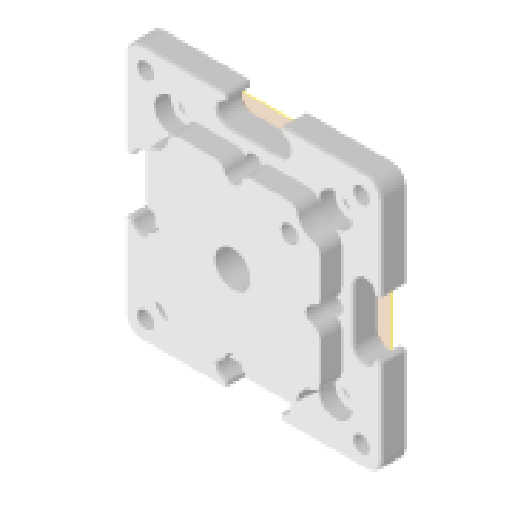
# Autodesk Inventor part: 40_XYZstage_micrometer_motorized_nema8_cube_ontop
Saved by Autodesk Inventor 2024.1 (Build 281209000, 209)
## iProperties
Created: 2023-06-28
Part Number: 40_XYZstage_micrometer_motorized_nema8_cube_ontop
Material: Generisch
Document SubType Name: Modeling
Designer: diederichbenedict
Density: 1 g/cm^3
Appearance: Vorgabe
Author: diederichbenedict
Autodesk Inventor part; units mm, degrees
ref_plane "YZ Plane" through (0, 0, 0) normal (1, 0, 0) x (0, 1, 0)
ref_plane "XZ Plane" through (0, 0, 0) normal (0, 1, 0) x (-1, 0, 0)
ref_plane "XY Plane" through (0, 0, 0) normal (0, 0, 1) x (1, 0, 0)
ref_plane "Arbeitsebene1" through (0, 0, 0) normal (0, 0, 1) x (1, 0, 0)
sketch "Skizze1" plane through (0, 0, 0) normal (0, 0, 1) x (1, 0, 0)
  line L0 (0, -40) -> (0, 0) projected
  line L1 (0, 0) -> (-40, 0) projected
  line L2 (-40, 0) -> (-40, -40) projected
  line L3 (-40, -40) -> (0, -40) projected
  circle A0 centre (-20, -20) radius 1.5 projected
  circle A1 centre (-4, -20) radius 1.5 projected
  circle A2 centre (-4, -4) radius 1.5 projected
  circle A3 centre (-20, -4) radius 1.5 projected
  circle A4 centre (-36, -4) radius 1.5 projected
  circle A5 centre (-36, -20) radius 1.5 projected
  circle A6 centre (-36, -36) radius 1.5 projected
  circle A7 centre (-20, -36) radius 1.5 projected
  circle A8 centre (-4, -36) radius 1.5 projected
  circle A9 centre (-9, -8.5) radius 1.5 projected
  line L4 (1.9, 4.9) -> (-41.9, 4.9)
  line L5 (-44.9, 1.9) -> (-44.9, -41.9)
  line L6 (-41.9, -44.9) -> (1.9, -44.9)
  line L7 (4.9, -41.9) -> (4.9, 1.9)
  line L8 (4.9, 4.9) -> (-44.9, -44.9) construction
  line L9 (-44.9, 4.9) -> (4.9, -44.9) construction
  arc A10 (-44.9, -41.9) -> (-41.9, -44.9) centre (-41.9, -41.9) ccw
  arc A11 (-41.9, 4.9) -> (-44.9, 1.9) centre (-41.9, 1.9) ccw
  arc A12 (4.9, 1.9) -> (1.9, 4.9) centre (1.9, 1.9) ccw
  arc A13 (1.9, -44.9) -> (4.9, -41.9) centre (1.9, -41.9) ccw
  line L10 (1, 1) -> (-41, 1) construction
  line L11 (-41, 1) -> (-41, -41) construction
  line L12 (-41, -41) -> (1, -41) construction
  line L13 (1, -41) -> (1, 1) construction
  line L14 (1, 1) -> (-41, -41) construction
  line L15 (-41, 1) -> (1, -41) construction
  circle A14 centre (-41, -41) radius 1.6
  circle A15 centre (1, 1) radius 1.6
  circle A16 centre (1, -41) radius 1.6
  circle A17 centre (-41, 1) radius 1.6
  point P0 (-40, -0.249)
  point P1 (-39.751, 0)
  dimension "d0" = 49.8
  dimension "d1" = 49.8
  dimension "d2" = 3
  dimension "d3" = 42
  dimension "d4" = 42
  dimension "d5" = 3.2
  dimension "d7" = 3.2
  dimension "d8" = 3.2
  dimension "d33" = 3.2
  constraints: 24 end point, 8 centre point, 8 point on circle, 8 point on line, 8 tangent, 4 coincident, 4 midpoint, 4 parallel, 3 equal radius, 2 horizontal, 2 perpendicular
  measures "d0" distance of L9.end L8.end
  measures "d1" distance of L8.end L9.start
  measures "d2" radius of A10
  measures "d3" distance of L12.end L11.end
  measures "d4" distance of L11.end L10.end
  measures "d5" diameter of A14
  measures "d7" diameter of A15
  measures "d8" diameter of A16
  measures "d33" diameter of A17
extrude "Extrusion1" add sketch "Skizze1" along normal blind 5 contours A16 L3 A14 L2 A17 L1 A15 L0 | A17 L2 L1 | A12 L7 A13 L6 A10 L5 A11 L4 picked at (-39.859606, -0.029677)
sketch "Skizze2" plane through (0, 0, 0) normal (0, 0, -1) x (-1, 0, 0)
  circle A0 centre (-1, -41) radius 1.6
  circle A1 centre (-1, 1) radius 1.6
  circle A2 centre (41, -41) radius 1.6
  line L0 (1.619086, -39.308732) -> (1.774224, -42.422562)
  line L1 (1.774224, -42.422562) -> (-0.844863, -44.113829)
  line L2 (-0.844863, -44.113829) -> (-3.619086, -42.691268)
  line L3 (-3.619086, -42.691268) -> (-3.774224, -39.577438)
  line L4 (-3.774224, -39.577438) -> (-1.155137, -37.886171)
  line L5 (-1.155137, -37.886171) -> (1.619086, -39.308732)
  line L6 (1.57078, -0.763828) -> (-1.24213, -2.108275)
  line L7 (-1.24213, -2.108275) -> (-3.81291, -0.344447)
  line L8 (-3.81291, -0.344447) -> (-3.57078, 2.763828)
  line L9 (-3.57078, 2.763828) -> (-0.75787, 4.108275)
  line L10 (-0.75787, 4.108275) -> (1.81291, 2.344447)
  line L11 (1.81291, 2.344447) -> (1.57078, -0.763828)
  line L12 (38.364164, -42.665043) -> (38.240113, -39.54982)
  line L13 (38.240113, -39.54982) -> (40.875949, -37.884777)
  line L14 (40.875949, -37.884777) -> (43.635836, -39.334957)
  line L15 (43.635836, -39.334957) -> (43.759887, -42.45018)
  line L16 (43.759887, -42.45018) -> (41.124051, -44.115223)
  line L17 (41.124051, -44.115223) -> (38.364164, -42.665043)
  line L18 (38.499173, -0.861683) -> (38.137322, 2.234938)
  line L19 (38.137322, 2.234938) -> (40.638149, 4.096621)
  line L20 (40.638149, 4.096621) -> (43.500827, 2.861683)
  line L21 (43.500827, 2.861683) -> (43.862678, -0.234938)
  line L22 (43.862678, -0.234938) -> (41.361851, -2.096621)
  line L23 (41.361851, -2.096621) -> (38.499173, -0.861683)
  arc A3 (40, -0.249) -> (39.751, 0) centre (41, 1) ccw
  point P0 (0, 0)
  dimension "d11" = 5.4
  dimension "d12" = 5.4
  dimension "d13" = 5.4
  dimension "d14" = 5.4
  constraints: 48 end point, 5 coincident, 52 other
  measures "d11" distance between parallel lines of L14 L17
  measures "d12" distance between parallel lines of L20 L23
  measures "d13" distance between parallel lines of L2 L5
  measures "d14" distance between parallel lines of L10 L7
extrude "Extrusion2" cut sketch "Skizze2" against normal blind 2.6 contours A0 | A1 | A2 | L0 L1 L2 L3 L4 L5 | L6 L7 L8 L9 L10 L11 | L12 L13 L14 L15 L16 L17 | L18 L19 L20 L21 L22 L23
sketch "Skizze3" plane through (0, 0, 5) normal (0, 0, 1) x (1, 0, 0)
  circle A0 centre (-36, -36) radius 1.5 projected
  circle A1 centre (-36, -4) radius 1.5 projected
  circle A2 centre (-4, -4) radius 1.5 projected
  circle A3 centre (-4, -36) radius 1.5 projected
  circle A4 centre (-20, -20) radius 1.5 projected
  point P0 (0, 0)
hole "Bohrung1" at (-36, -4, 5) at (-4, -4, 5) at (-4, -36, 5) at (-36, -36, 5) at (-20, -20, 5) direction (0, 0, -1) diameter 3.2 end through all counterbore diameter 6.5 counterbore depth 3
sketch "Skizze4" plane through (0, 0, 5) normal (0, 0, 1) x (1, 0, 0)
  arc A0 (-43.37115, -25.66459) -> (-39.55, -25.05) centre (-41.51, -25.05) ccw
  arc A1 (-43.37115, -25.66459) -> (-44.083261, -25.149765) centre (-44.083325, -25.899765) ccw
  line L0 (-44.083261, -25.149765) -> (-45, -25.149687)
  line L1 (-39.55, -14.95) -> (-39.55, -25.05)
  arc A2 (-39.55, -14.95) -> (-43.37115, -14.33541) centre (-41.51, -14.95) ccw
  arc A3 (-44.083261, -14.850235) -> (-43.37115, -14.33541) centre (-44.083325, -14.100235) ccw
  arc A4 (-45, -14.100249) -> (-44.249937, -14.850249) centre (-44.25, -14.100249) ccw
  line L2 (-44.249937, -14.850249) -> (-44.083261, -14.850235)
  line L3 (-45, -25.149687) -> (-45, -43)
  line L4 (-45, 3) -> (-45, -14.100249)
  line L5 (-45, -25.999984) -> (-45, -14.100249)
  line L6 (-44.9, 1.9) -> (-44.9, -41.9)
  line L7 (-44.9, -43) -> (-44.9, -25.249696)
  line L8 (-44.9, -25.249696) -> (-44.08327, -25.249765)
  arc A5 (-43.466107, -25.695947) -> (-44.08327, -25.249765) centre (-44.083325, -25.899765) ccw
  arc A6 (-43.466107, -25.695947) -> (-39.45, -25.05) centre (-41.51, -25.05) ccw
  line L9 (-39.45, -25.05) -> (-39.45, -14.95)
  arc A7 (-39.45, -14.95) -> (-43.466107, -14.304053) centre (-41.51, -14.95) ccw
  arc A8 (-44.08327, -14.750235) -> (-43.466107, -14.304053) centre (-44.083325, -14.100235) ccw
  line L10 (-44.08327, -14.750235) -> (-44.249945, -14.750249)
  arc A9 (-44.9, -14.100249) -> (-44.249945, -14.750249) centre (-44.25, -14.100249) ccw
  line L11 (-44.9, -14.100249) -> (-44.9, 3)
  arc A10 (-44.25, -25.249751) -> (-45, -25.999984) centre (-44.051013, -26.198676) ccw
  point P0 (0, 0)
  point P1 (-44.9, -14.474415)
  dimension "d24" = 0.1
  constraints: 12 end point, 12 point on circle, 6 centre point, 2 point on line, 1 parallel, 9 other
  measures "d24" radial gap between concentric circles of A1 A5
extrude "Extrusion3" cut sketch "Skizze4" against normal through all
pattern_circular "Runde Anordnung1" count 4 over 360 about axis through (-20, -20, 0) along (0, 0, 1) of "Extrusion3"
chamfer "Fase1" distance 0.3 angle 45 88 edges at (-44.9, -33.8152, 5) (-44.0213, -44.0213, 5) (-33.8999, -44.9, 5) (-25.4401, -44.7096, 5) (-25.2498, -44.1666, 5) (-25.373, -43.7025, 5) (-27.0839, -41.1829, 5) (-20, -39.45, 5) (-12.9161, -41.1829, 5) (-14.627, -43.7025, 5) (-14.7502, -44.1666, 5) (-41.1829, -27.0839, 5) (-43.7025, -25.373, 5) (-44.1666, -25.2498, 5) (-39.45, -20, 5) (-41.1829, -12.9161, 5) (-43.7025, -14.627, 5) (-44.1666, -14.7502, 5) (-44.7096, -14.5599, 5) (-44.9, -6.1001, 5) (-44.0213, 4.0213, 5) (-33.8152, 4.9, 5) (-6.1848, -44.9, 5) (4.0213, -44.0213, 5) (4.9, -33.8999, 5) (4.7096, -25.4401, 5) (4.1666, -25.2498, 5) (3.7025, -25.373, 5) (1.1829, -27.0839, 5) (-0.55, -20, 5) (1.1829, -12.9161, 5) (3.7025, -14.627, 5) (4.1666, -14.7502, 5) (-12.9161, 1.1829, 5) (-20, -0.55, 5) (-27.0839, 1.1829, 5) (-25.373, 3.7025, 5) (-25.2498, 4.1666, 5) (-14.627, 3.7025, 5) (-14.7502, 4.1666, 5) (-14.5599, 4.7096, 5) (-6.1001, 4.9, 5) (4.0213, 4.0213, 5) (4.9, -6.1848, 5) (4.9, -33.8999, 0) (4.7096, -25.4401, 0) (4.1666, -25.2498, 0) (3.7025, -25.373, 0) (1.1829, -27.0839, 0) (-0.55, -20, 0) (1.1829, -12.9161, 0) (3.7025, -14.627, 0) (4.1666, -14.7502, 0) (4.0213, -44.0213, 0) (-6.1848, -44.9, 0) (4.9, -6.1848, 0) (4.0213, 4.0213, 0) (-6.1001, 4.9, 0) (-14.5599, 4.7096, 0) (-14.7502, 4.1666, 0) (-14.627, 3.7025, 0) (-12.9161, 1.1829, 0) (-20, -0.55, 0) (-27.0839, 1.1829, 0) (-25.373, 3.7025, 0) (-25.2498, 4.1666, 0) (-33.8152, 4.9, 0) (-44.9, -6.1001, 0) (-44.7096, -14.5599, 0) (-44.1666, -14.7502, 0) (-43.7025, -14.627, 0) (-41.1829, -12.9161, 0) (-39.45, -20, 0) (-41.1829, -27.0839, 0) (-43.7025, -25.373, 0) (-44.1666, -25.2498, 0) (-44.0213, 4.0213, 0) (-44.9, -33.8152, 0) (-44.0213, -44.0213, 0) (-33.8999, -44.9, 0) (-25.4401, -44.7096, 0) (-25.2498, -44.1666, 0) (-25.373, -43.7025, 0) (-27.0839, -41.1829, 0) (-20, -39.45, 0) (-12.9161, -41.1829, 0) (-14.627, -43.7025, 0) (-14.7502, -44.1666, 0)
sketch "Skizze5" plane through (0, 0, 5) normal (0, 0, 1) x (1, 0, 0)
  circle A0 centre (1, 1) radius 1.6
  circle A1 centre (-4, -20) radius 1.5
  circle A2 centre (-20, -4) radius 1.5
  circle A3 centre (-36, -20) radius 1.5
  circle A4 centre (-20, -36) radius 1.5
  circle A5 centre (-9, -8.5) radius 1.5
  circle A6 centre (1, -41) radius 1.6
  circle A7 centre (-41, -41) radius 1.6
  arc A8 (-39.751, 0) -> (-40, -0.249) centre (-41, 1) ccw
  line L0 (-39.751, 0) -> (-40, 0)
  line L1 (-40, 0) -> (-40, -0.249)
  circle A9 centre (-36, -36) radius 3.25
  circle A10 centre (-4, -4) radius 3.25
  circle A11 centre (-36, -4) radius 3.25
  circle A12 centre (-4, -36) radius 3.25
  line L2 (4.6, 1.9) -> (4.6, -14.450279)
  arc A13 (4.6, 1.9) -> (1.9, 4.6) centre (1.9, 1.9) ccw
  line L3 (-14.100249, 4.6) -> (1.9, 4.6)
  arc A14 (-14.100249, 4.6) -> (-14.450249, 4.24997) centre (-14.100249, 4.25) ccw
  line L4 (-14.450235, 4.083295) -> (-14.450249, 4.24997)
  arc A15 (-14.450235, 4.083295) -> (-14.209984, 3.750977) centre (-14.100235, 4.083325) ccw
  arc A16 (-14.95, -0.85) -> (-14.209984, 3.750977) centre (-14.95, 1.51) ccw
  line L5 (-25.05, -0.85) -> (-14.95, -0.85)
  arc A17 (-25.790016, 3.750977) -> (-25.05, -0.85) centre (-25.05, 1.51) ccw
  arc A18 (-25.790016, 3.750977) -> (-25.549765, 4.083295) centre (-25.899765, 4.083325) ccw
  line L6 (-25.549721, 4.6) -> (-25.549765, 4.083295)
  line L7 (-41.9, 4.6) -> (-25.549721, 4.6)
  arc A19 (-41.9, 4.6) -> (-44.6, 1.9) centre (-41.9, 1.9) ccw
  line L8 (-44.6, -14.100249) -> (-44.6, 1.9)
  arc A20 (-44.6, -14.100249) -> (-44.24997, -14.450249) centre (-44.25, -14.100249) ccw
  line L9 (-44.083295, -14.450235) -> (-44.24997, -14.450249)
  arc A21 (-44.083295, -14.450235) -> (-43.750977, -14.209984) centre (-44.083325, -14.100235) ccw
  arc A22 (-39.15, -14.95) -> (-43.750977, -14.209984) centre (-41.51, -14.95) ccw
  line L10 (-39.15, -25.05) -> (-39.15, -14.95)
  arc A23 (-43.750977, -25.790016) -> (-39.15, -25.05) centre (-41.51, -25.05) ccw
  arc A24 (-43.750977, -25.790016) -> (-44.083295, -25.549765) centre (-44.083325, -25.899765) ccw
  line L11 (-44.6, -25.549721) -> (-44.083295, -25.549765)
  line L12 (-44.6, -41.9) -> (-44.6, -25.549721)
  arc A25 (-44.6, -41.9) -> (-41.9, -44.6) centre (-41.9, -41.9) ccw
  line L13 (-25.899751, -44.6) -> (-41.9, -44.6)
  arc A26 (-25.899751, -44.6) -> (-25.549751, -44.24997) centre (-25.899751, -44.25) ccw
  line L14 (-25.549765, -44.083295) -> (-25.549751, -44.24997)
  arc A27 (-25.549765, -44.083295) -> (-25.790016, -43.750977) centre (-25.899765, -44.083325) ccw
  arc A28 (-25.05, -39.15) -> (-25.790016, -43.750977) centre (-25.05, -41.51) ccw
  line L15 (-14.95, -39.15) -> (-25.05, -39.15)
  arc A29 (-14.209984, -43.750977) -> (-14.95, -39.15) centre (-14.95, -41.51) ccw
  arc A30 (-14.209984, -43.750977) -> (-14.450235, -44.083295) centre (-14.100235, -44.083325) ccw
  line L16 (-14.450279, -44.6) -> (-14.450235, -44.083295)
  line L17 (1.9, -44.6) -> (-14.450279, -44.6)
  arc A31 (1.9, -44.6) -> (4.6, -41.9) centre (1.9, -41.9) ccw
  line L18 (4.6, -25.899751) -> (4.6, -41.9)
  arc A32 (4.6, -25.899751) -> (4.24997, -25.549751) centre (4.25, -25.899751) ccw
  line L19 (4.083295, -25.549765) -> (4.24997, -25.549751)
  arc A33 (4.083295, -25.549765) -> (3.750977, -25.790016) centre (4.083325, -25.899765) ccw
  arc A34 (-0.85, -25.05) -> (3.750977, -25.790016) centre (1.51, -25.05) ccw
  line L20 (-0.85, -14.95) -> (-0.85, -25.05)
  arc A35 (3.750977, -14.209984) -> (-0.85, -14.95) centre (1.51, -14.95) ccw
  arc A36 (3.750977, -14.209984) -> (4.083295, -14.450235) centre (4.083325, -14.100235) ccw
  line L21 (4.6, -14.450279) -> (4.083295, -14.450235)
  line L22 (-37.2, -37.2) -> (-2.8, -37.2)
  line L23 (-2.8, -37.2) -> (-2.8, -2.8)
  line L24 (-2.8, -2.8) -> (-37.2, -2.8)
  line L25 (-37.2, -2.8) -> (-37.2, -37.2)
  circle A37 centre (-20, -20) radius 1.5
  line L26 (-37.2, -37.2) -> (-2.8, -2.8) construction
  line L27 (-2.8, -37.2) -> (-37.2, -2.8) construction
  circle A38 centre (-20, -20) radius 3.25
  point P0 (0, 0)
  point P1 (-37.2, -20.9)
  point P2 (-37.2, -32.979652)
  point P3 (-32.979652, -37.2)
  point P4 (-20.9, -37.2)
  point P5 (-19.1, -37.2)
  point P6 (-7.020348, -37.2)
  point P7 (-2.8, -32.979652)
  point P8 (-2.8, -20.9)
  point P9 (-2.8, -19.1)
  point P10 (-2.8, -7.020348)
  point P11 (-7.020348, -2.8)
  point P12 (-19.1, -2.8)
  point P13 (-20.9, -2.8)
  point P14 (-32.979652, -2.8)
  point P15 (-37.2, -7.020348)
  point P16 (-37.2, -19.1)
  dimension "d34" = 34.4
  dimension "d35" = 34.4
  constraints: 12 end point, 2 midpoint, 2 parallel, 1 horizontal, 1 perpendicular
  measures "d34" distance of L24.end L23.end
  measures "d35" distance of L23.end L22.end
extrude "Extrusion4" add sketch "Skizze5" along normal blind 4 draft -3 contours A1 L23 A12 L22 A4 A9 L25 A3 A11 L24 A2 A10
fillet "Rundung1" radius 2 16 edges at (-7.1676, -2.9024, 6.9535) (-2.9024, -7.1676, 6.9535) (-2.8935, -21.1468, 6.7848) (-2.8935, -18.8532, 6.7848) (-2.9024, -32.8324, 6.9535) (-7.1676, -37.0976, 6.9535) (-18.8532, -37.1065, 6.7848) (-21.1468, -37.1065, 6.7848) (-32.8324, -37.0976, 6.9535) (-37.0976, -32.8324, 6.9535) (-37.1065, -21.1468, 6.7848) (-37.1065, -18.8532, 6.7848) (-37.0976, -7.1676, 6.9535) (-32.8324, -2.9024, 6.9535) (-21.1468, -2.8935, 6.7848) (-18.8532, -2.8935, 6.7848)
equation "\"d12\" = d11"
equation "\"d13\" = d11"
equation "\"d14\" = d11"
